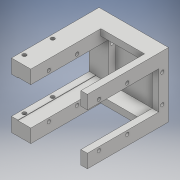
# Autodesk Inventor part: elbow_fore
Saved by Autodesk Inventor 2018 (Build 220112000, 112)
## iProperties
Created: 2020-09-08
Part Number: elbow_fore
Material: 일반
Document SubType Name: Modeling
Designer: j3jjj
Density: 1 g/cm^3
Appearance: 기본값
Author: j3jjj
Autodesk Inventor part; units mm, degrees
ref_plane "YZ Plane" through (0, 0, 0) normal (1, 0, 0) x (0, 1, 0)
ref_plane "XZ Plane" through (0, 0, 0) normal (0, 1, 0) x (-1, 0, 0)
ref_plane "XY Plane" through (0, 0, 0) normal (0, 0, 1) x (1, 0, 0)
sketch "스케치1" plane through (0, 0, 0) normal (0, 1, 0) x (-1, 0, 0)
  line L0 (22, -14) -> (-22, -14)
  line L1 (-22, -14) -> (-22, 14)
  line L2 (-22, 14) -> (22, 14)
  line L3 (22, 14) -> (22, -14)
  point P0 (0, 0)
  dimension "d0" = 44
  dimension "d1" = 22
  dimension "d2" = 28
  dimension "d3" = 14
  constraints: 8 end point, 2 parallel, 1 horizontal, 1 perpendicular
  measures "d0" distance between parallel lines of L1 L3
  measures "d1" distance from line of point (0, 0) L3
  measures "d2" distance between parallel lines of L0 L2
  measures "d3" distance from line of point (0, 0) L0
extrude "돌출1" add sketch "스케치1" along normal blind 5
sketch "스케치2" plane through (-22, 0, 14) normal (0, 0, 1) x (1, 0, 0)
  circle A0 centre (33, 3) radius 1.5
  circle A1 centre (11, 3) radius 1.5
  line L0 (44, 0) -> (0, 0) projected
  line L1 (22, 0) -> (22, 5)
  line L2 (44, 5) -> (0, 5) projected
  dimension "d6" = 3
  dimension "d7" = 3
  dimension "d8" = 3
  dimension "d9" = 3
  dimension "d10" = 22
  dimension "d11" = 11
  constraints: 2 centre point, 2 end point, 1 midpoint
  measures "d6" diameter of A1
  measures "d7" diameter of A0
  measures "d8" distance from line of A0.centre L0
  measures "d9" distance from line of L0 A1.centre
  measures "d10" distance of A0.centre A1.centre
  measures "d11" distance from line of L1 A1.centre
extrude "돌출2" cut sketch "스케치2" against normal blind 60
sketch "스케치3" plane through (0, 0, 0) normal (0, -1, 0) x (1, 0, 0)
  line L0 (-17, 14.5) -> (17, 14.5)
  line L1 (17, 14.5) -> (17, -14.5)
  line L2 (17, -14.5) -> (-17, -14.5)
  line L3 (-17, -14.5) -> (-17, 14.5)
  line L4 (22, -14) -> (-22, -14) projected
  line L5 (22, 25.1) -> (-22, 25.1)
  line L6 (-22, 25.1) -> (-22, -25.1)
  line L7 (-22, -25.1) -> (22, -25.1)
  line L8 (22, -25.1) -> (22, 25.1)
  point P0 (0, 0)
  dimension "d17" = 34
  dimension "d18" = 17
  dimension "d20" = 29
  dimension "d21" = 14.5
  dimension "d22" = 10.6
  dimension "d23" = 10.6
  dimension "d24" = 5
  dimension "d25" = 5
  constraints: 16 end point, 4 parallel, 2 horizontal, 2 perpendicular
  measures "d17" distance between parallel lines of L1 L3
  measures "d18" distance from line of point (0, 0) L3
  measures "d20" distance between parallel lines of L2 L0
  measures "d21" distance from line of point (0, 0) L0
  measures "d22" distance between parallel lines of L0 L5
  measures "d23" distance between parallel lines of L7 L2
  measures "d24" distance between parallel lines of L8 L1
  measures "d25" distance between parallel lines of L3 L6
extrude "돌출3" add sketch "스케치3" along normal blind 2
sketch "스케치4" plane through (0, -2, 0) normal (0, -1, 0) x (1, 0, 0)
  line L0 (-22, 25.1) -> (-22, -25.1) projected
  line L1 (-22, -25.1) -> (22, -25.1) projected
  line L2 (-22, 25.1) -> (22, 25.1)
  line L3 (22, 25.1) -> (22, -25.1)
  line L4 (22, -25.1) -> (-22, -25.1)
  line L5 (-22, -25.1) -> (-22, 25.1)
  line L6 (-17, 20.1) -> (17, 20.1)
  line L7 (17, 20.1) -> (17, -20.1)
  line L8 (17, -20.1) -> (-17, -20.1)
  line L9 (-17, -20.1) -> (-17, 20.1)
  point P0 (0, 0)
  dimension "d28" = 5
  dimension "d29" = 5
  dimension "d30" = 5
  dimension "d31" = 5
  constraints: 16 end point, 4 parallel, 2 horizontal, 2 perpendicular
  measures "d28" distance between parallel lines of L6 L2
  measures "d29" distance between parallel lines of L1 L8
  measures "d30" distance between parallel lines of L9 L0
  measures "d31" distance between parallel lines of L3 L7
extrude "돌출4" add sketch "스케치4" along normal blind 5.58
sketch "스케치5" plane through (22, 5, 14) normal (1, 0, 0) x (0, 0, -1)
  circle A0 centre (25, -9.8) radius 1.35
  circle A1 centre (3, -9.8) radius 1.35
  line L0 (39.1, -5) -> (28, -5) projected
  line L1 (0, -5) -> (-11.1, -5) projected
  point P0 (14, -5)
  dimension "d34" = 2.7
  dimension "d35" = 2.7
  dimension "d36" = 4.8
  dimension "d37" = 4.8
  dimension "d38" = 22
  dimension "d39" = 11
  constraints: 2 centre point
  measures "d34" diameter of A0
  measures "d35" diameter of A1
  measures "d36" distance from line of A0.centre L0
  measures "d37" distance from line of A1.centre L1
  measures "d38" distance of A1.centre A0.centre
  measures "d39" horizontal distance of point (14, -5) A0.centre
extrude "돌출5" cut sketch "스케치5" against normal blind 90
sketch "스케치6" plane through (0, -7.58, 0) normal (0, -1, 0) x (1, 0, 0)
  line L0 (22, -25.1) -> (-22, -25.1)
  line L1 (-22, -25.1) -> (-22, -20.1)
  line L2 (-22, -20.1) -> (22, -20.1)
  line L3 (22, -20.1) -> (22, -25.1)
  line L4 (22, 25.1) -> (-22, 25.1)
  line L5 (-22, 25.1) -> (-22, 20.1)
  line L6 (-22, 20.1) -> (22, 20.1)
  line L7 (22, 20.1) -> (22, 25.1)
  point P0 (0, 0)
  dimension "d42" = 5
  dimension "d43" = 5
  constraints: 16 end point, 4 parallel, 2 horizontal, 2 perpendicular
  measures "d42" distance between parallel lines of L2 L0
  measures "d43" distance between parallel lines of L4 L6
extrude "돌출6" add sketch "스케치6" along normal blind 6
sketch "스케치7" plane through (0, -7.58, 0) normal (0, -1, 0) x (1, 0, 0)
  line L0 (22, -20.1) -> (-22, -20.1) projected
  line L1 (17, 20.1) -> (17, -20.1) projected
  line L2 (22, -20.1) -> (17, -20.1)
  line L3 (17, -20.1) -> (17, -14.6)
  line L4 (17, -14.6) -> (22, -14.6)
  line L5 (22, -14.6) -> (22, -20.1)
  line L6 (22, 14) -> (22, 25.1) projected
  line L7 (22, 20.1) -> (17, 20.1)
  line L8 (17, 20.1) -> (17, 14.6)
  line L9 (17, 14.6) -> (22, 14.6)
  line L10 (22, 14.6) -> (22, 20.1)
  line L11 (-22, -14) -> (-22, 14) projected
  line L12 (-17, -20.1) -> (-22, -20.1)
  line L13 (-22, -20.1) -> (-22, -14.6)
  line L14 (-22, -14.6) -> (-17, -14.6)
  line L15 (-17, -14.6) -> (-17, -20.1)
  line L16 (-17, 20.1) -> (-22, 20.1)
  line L17 (-22, 20.1) -> (-22, 14.6)
  line L18 (-22, 14.6) -> (-17, 14.6)
  line L19 (-17, 14.6) -> (-17, 20.1)
  line L20 (22, 20.1) -> (17, 20.1) projected
  point P0 (0, 0)
  dimension "d46" = 5.5
  dimension "d47" = 5.5
  dimension "d48" = 5.5
  dimension "d49" = 5.5
  dimension "d50" = 0
  constraints: 32 end point, 8 parallel, 5 point on line, 4 horizontal, 4 perpendicular
  measures "d46" distance between parallel lines of L4 L0
  measures "d47" distance between parallel lines of L7 L9
  measures "d48" distance between parallel lines of L14 L0
  measures "d49" distance between parallel lines of L16 L18
  measures "d50" distance between parallel lines of L20 L7
extrude "돌출7" add sketch "스케치7" along normal blind 55.52
sketch "스케치8" plane through (0, -13.58, 0) normal (0, -1, 0) x (1, 0, 0)
  line L0 (-22, -20.1) -> (-22, -25.1) projected
  line L1 (-17, -20.1) -> (-22, -20.1) projected
  line L2 (-22, -25.1) -> (-17, -25.1)
  line L3 (-17, -25.1) -> (-17, -20.1)
  line L4 (-17, -20.1) -> (-22, -20.1)
  line L5 (-22, -20.1) -> (-22, -25.1)
  line L6 (-17, -20.1) -> (17, -20.1) projected
  line L7 (22, -25.1) -> (22, -20.1) projected
  line L8 (17, -20.1) -> (22, -20.1)
  line L9 (22, -20.1) -> (22, -25.1)
  line L10 (22, -25.1) -> (17, -25.1)
  line L11 (17, -25.1) -> (17, -20.1)
  line L12 (17, -20.1) -> (17, 20.1) projected
  line L13 (22, 20.1) -> (22, 25.1) projected
  line L14 (17, 20.1) -> (22, 20.1)
  line L15 (22, 20.1) -> (22, 25.1)
  line L16 (22, 25.1) -> (17, 25.1)
  line L17 (17, 25.1) -> (17, 20.1)
  line L18 (-22, 25.1) -> (-22, 20.1) projected
  line L19 (22, 25.1) -> (-22, 25.1) projected
  line L20 (-22, 20.1) -> (-17, 20.1)
  line L21 (-17, 20.1) -> (-17, 25.1)
  line L22 (-17, 25.1) -> (-22, 25.1)
  line L23 (-22, 25.1) -> (-22, 20.1)
  point P0 (0, 0)
  constraints: 32 end point, 8 parallel, 4 horizontal, 4 perpendicular, 2 point on line
extrude "돌출8" add sketch "스케치8" along normal blind 49.52
sketch "스케치9" plane through (-22, 5, -14) normal (-1, 0, 0) x (0, 0, 1)
  circle A0 centre (31.3, -59.1) radius 1.35
  circle A1 centre (-3.3, -59.1) radius 1.35
  line L0 (-0.6, -68.1) -> (-11.1, -68.1) projected
  line L1 (39.1, -68.1) -> (28.6, -68.1) projected
  line L2 (39.1, -5) -> (39.1, -68.1) projected
  line L3 (-11.1, -5) -> (-11.1, -68.1) projected
  circle A2 centre (31.3, -37.1) radius 1.35
  circle A3 centre (-3.3, -37.1) radius 1.35
  point P0 (14, -5)
  dimension "d55" = 9
  dimension "d56" = 9
  dimension "d57" = 2.7
  dimension "d58" = 2.7
  dimension "d59" = 7.8
  dimension "d60" = 7.8
  dimension "d61" = 2.7
  dimension "d62" = 2.7
  dimension "d63" = 22
  dimension "d64" = 22
  constraints: 4 centre point
  measures "d55" distance from line of A1.centre L0
  measures "d56" distance from line of A0.centre L1
  measures "d57" diameter of A0
  measures "d58" diameter of A1
  measures "d59" distance from line of A0.centre L2
  measures "d60" distance from line of A1.centre L3
  measures "d61" diameter of A3
  measures "d62" diameter of A2
  measures "d63" distance of A3.centre A1.centre
  measures "d64" distance of A2.centre A0.centre
extrude "돌출9" cut sketch "스케치9" against normal blind 49.52
sketch "스케치11" plane through (-22, 5, -14) normal (-1, 0, 0) x (0, 0, 1)
  line L0 (28, 0) -> (0, 0) projected
  line L1 (0, -5) -> (-11.1, -5) projected
  line L2 (28, 0) -> (0, 0)
  line L3 (0, 0) -> (0, -5)
  line L4 (0, -5) -> (28, -5)
  line L5 (28, -5) -> (28, 0)
  point P0 (14, -5)
  constraints: 8 end point, 2 parallel, 1 horizontal, 1 perpendicular
extrude "돌출11" cut sketch "스케치11" against normal blind 80
sketch "스케치14" plane through (-22, 0, -25.1) normal (-1, 0, 0) x (0, 0, 1)
  line L0 (0, -63.1) -> (10.5, -63.1) projected
  line L1 (0, -63.1) -> (10.5, -63.1)
  line L2 (10.5, -7.58) -> (10.5, -63.1) projected
  line L3 (10.5, -63.1) -> (10.5, -7.58)
  line L4 (10.5, -7.58) -> (39.7, -7.58)
  line L5 (39.7, -7.58) -> (39.7, -63.1) projected
  line L6 (39.7, -7.58) -> (39.7, -63.1)
  line L7 (39.7, -63.1) -> (50.2, -63.1) projected
  line L8 (39.7, -63.1) -> (50.2, -63.1)
  line L9 (50.2, 0) -> (50.2, -63.1) projected
  line L10 (50.2, -63.1) -> (50.2, 0)
  line L11 (50.2, 0) -> (0, 0) projected
  line L12 (50.2, 0) -> (0, 0)
  line L13 (0, -13.58) -> (0, -63.1) projected
  line L14 (0, 0) -> (0, -63.1)
  point P0 (25.1, 0)
  constraints: 16 end point, 5 perpendicular, 3 collinear
extrude "돌출14" add sketch "스케치14" along normal blind 10
sketch "스케치15" plane through (-17, -63.1, 14.6) normal (0, 0, -1) x (-1, 0, 0)
  line L0 (15, 55.52) -> (15, 0) projected
  line L1 (0, 55.52) -> (15, 55.52) projected
  line L2 (15, 0) -> (10, 0)
  line L3 (10, 0) -> (10, 55.52)
  line L4 (10, 55.52) -> (15, 55.52)
  line L5 (15, 55.52) -> (15, 0)
  point P0 (-17, 63.1)
  dimension "d86" = 5
  constraints: 8 end point, 2 parallel, 1 horizontal, 1 perpendicular, 1 point on line
  measures "d86" distance between parallel lines of L0 L3
extrude "돌출15" add sketch "스케치15" along normal blind 0.4
sketch "스케치16" plane through (-17, -63.1, -14.6) normal (0, 0, 1) x (1, 0, 0)
  line L0 (-15, 0) -> (-15, 55.52) projected
  line L1 (-15, 55.52) -> (0, 55.52) projected
  line L2 (-15, 0) -> (-10, 0)
  line L3 (-10, 0) -> (-10, 55.52)
  line L4 (-10, 55.52) -> (-15, 55.52)
  line L5 (-15, 55.52) -> (-15, 0)
  point P0 (17, 63.1)
  dimension "d89" = 5
  constraints: 8 end point, 2 parallel, 1 horizontal, 1 perpendicular, 1 point on line
  measures "d89" distance between parallel lines of L0 L3
extrude "돌출16" add sketch "스케치16" along normal blind 0.4
sketch "스케치17" plane through (17, -13.58, -25.1) normal (0, 0, -1) x (-1, 0, 0)
  line L0 (13.776, -36.52) -> (66.3511, -36.52)
  line L1 (34, -49.52) -> (49, -49.52) projected
  circle A0 centre (46, -47.52) radius 1.5
  circle A1 centre (46, -25.52) radius 1.5
  line L2 (49, 13.58) -> (49, -49.52) projected
  point P0 (17, 13.58)
  dimension "d92" = 13
  dimension "d93" = 3
  dimension "d94" = 3
  dimension "d95" = 3
  dimension "d96" = 3
  dimension "d97" = 22
  dimension "d98" = 11
  constraints: 2 centre point, 2 end point, 1 horizontal
  measures "d92" distance between parallel lines of L0 L1
  measures "d93" diameter of A0
  measures "d94" diameter of A1
  measures "d95" distance from line of L2 A0.centre
  measures "d96" distance from line of L2 A1.centre
  measures "d97" distance of A1.centre A0.centre
  measures "d98" distance from line of L0 A0.centre
extrude "돌출17" cut sketch "스케치17" against normal blind 100
sketch "스케치18" plane through (0, -63.1, 0) normal (0, -1, 0) x (1, 0, 0)
  line L0 (-17, 25.1) -> (-17, 20.1) projected
  line L1 (-17, 14.6) -> (-27, 14.6) projected
  line L2 (-17, 25.1) -> (-27, 25.1)
  line L3 (-27, 25.1) -> (-27, 14.6)
  line L4 (-27, 14.6) -> (-17, 14.6)
  line L5 (-17, 14.6) -> (-17, 25.1)
  line L6 (-27, 14.2) -> (-32, 14.2) projected
  line L7 (-27, 25.1) -> (-32, 25.1)
  line L8 (-32, 25.1) -> (-32, 14.2)
  line L9 (-32, 14.2) -> (-27, 14.2)
  line L10 (-27, 14.2) -> (-27, 25.1)
  line L11 (-27, -14.6) -> (-17, -14.6) projected
  line L12 (22, -25.1) -> (-32, -25.1) projected
  line L13 (-17, -14.6) -> (-27, -14.6)
  line L14 (-27, -14.6) -> (-27, -25.1)
  line L15 (-27, -25.1) -> (-17, -25.1)
  line L16 (-17, -25.1) -> (-17, -14.6)
  line L17 (-32, -14.2) -> (-27, -14.2) projected
  line L18 (-32, 25.1) -> (-32, -25.1) projected
  line L19 (-27, -14.2) -> (-32, -14.2)
  line L20 (-32, -14.2) -> (-32, -25.1)
  line L21 (-32, -25.1) -> (-27, -25.1)
  line L22 (-27, -25.1) -> (-27, -14.2)
  point P0 (0, 0)
  constraints: 32 end point, 8 parallel, 4 horizontal, 4 perpendicular, 2 point on line
extrude "돌출18" add sketch "스케치18" along normal blind 5
